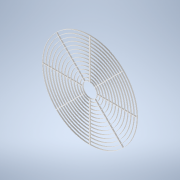
# Autodesk Inventor part: GitterUnten
Saved by Autodesk Inventor 2020.3 (Build 243373000, 373)
## iProperties
Created: 2020-08-06
Part Number: GitterUnten
Material: Generisch
Document SubType Name: Modeling
Designer: Stefan
Density: 1 g/cm^3
Appearance: Vorgabe
Author: Stefan
Autodesk Inventor part; units mm, degrees
ref_plane "YZ Plane" through (0, 0, 0) normal (1, 0, 0) x (0, 1, 0)
ref_plane "XZ Plane" through (0, 0, 0) normal (0, 1, 0) x (-1, 0, 0)
ref_plane "XY Plane" through (0, 0, 0) normal (0, 0, 1) x (1, 0, 0)
sketch "Skizze1" plane through (0, 0, 0) normal (0, 0, 1) x (1, 0, 0)
  line L0 (-278.3282, -259.073) -> (-259.0817, -278.3194) construction
  line L1 (-46.0536, -35.2636) -> (-10.8976, -70.4197) construction
  line L2 (-57.4999, 19.1327) -> (-57.4999, -6.5211) construction
  line L3 (-49.3128, 32.0045) -> (-8.1395, 73.1778) construction
  line L4 (-2, -377.9947) -> (-2, -354.9944)
  line L5 (-2, -352.9943) -> (-2, -329.9939)
  line L6 (-2, -327.9939) -> (-2, -304.9934)
  line L7 (-2, -302.9934) -> (-2, -279.9929)
  line L8 (-2, -277.9928) -> (-2, -254.9922)
  line L9 (-2, -252.9921) -> (-2, -229.9913)
  line L10 (-2, -227.9912) -> (-2, -204.9902)
  line L11 (-2, -202.9902) -> (-2, -179.9889)
  line L12 (-2, -177.9888) -> (-2, -154.9871)
  line L13 (-2, -152.9869) -> (-2, -129.9846)
  line L14 (-2, -127.9844) -> (-2, -104.981)
  line L15 (-2, -102.9806) -> (-2, -79.975)
  line L16 (-2, -77.9744) -> (-2, -59.4664)
  arc A0 (-265.8684, -268.6968) -> (-2, -377.9947) centre (0, 0) ccw
  arc A1 (-249.6047, -252.4331) -> (-2, -354.9944) centre (0, 0) ccw
  arc A2 (-248.1905, -251.0189) -> (-2, -352.9943) centre (0, 0) ccw
  line L17 (-252.4331, -249.6047) -> (-268.6968, -265.8684)
  line L18 (-265.8684, -268.6968) -> (-249.6047, -252.4331)
  arc A3 (-214.2487, -217.0771) -> (-2, -304.9934) centre (0, 0) ccw
  arc A4 (-212.8345, -215.6629) -> (-2, -302.9934) centre (0, 0) ccw
  arc A5 (-196.5706, -199.3991) -> (-2, -279.9929) centre (0, 0) ccw
  arc A6 (-178.8925, -181.7209) -> (-2, -254.9922) centre (0, 0) ccw
  arc A7 (-177.4782, -180.3066) -> (-2, -252.9921) centre (0, 0) ccw
  arc A8 (-161.2142, -164.0426) -> (-2, -229.9913) centre (0, 0) ccw
  arc A9 (-159.7999, -162.6284) -> (-2, -227.9912) centre (0, 0) ccw
  arc A10 (-143.5358, -146.3642) -> (-2, -204.9902) centre (0, 0) ccw
  arc A11 (-142.1215, -144.9499) -> (-2, -202.9902) centre (0, 0) ccw
  arc A12 (-231.9267, -234.7552) -> (-2, -329.9939) centre (0, 0) ccw
  arc A13 (-230.5125, -233.3409) -> (-2, -327.9939) centre (0, 0) ccw
  line L19 (-234.7552, -231.9267) -> (-251.0189, -248.1905)
  line L20 (-248.1905, -251.0189) -> (-231.9267, -234.7552)
  line L21 (-217.0771, -214.2487) -> (-233.3409, -230.5125)
  line L22 (-230.5125, -233.3409) -> (-214.2487, -217.0771)
  line L23 (-199.3991, -196.5706) -> (-215.6629, -212.8345)
  arc A14 (-195.1564, -197.9848) -> (-2, -277.9928) centre (0, 0) ccw
  line L24 (-212.8345, -215.6629) -> (-196.5706, -199.3991)
  line L25 (-181.7209, -178.8925) -> (-197.9848, -195.1564)
  line L26 (-195.1564, -197.9848) -> (-178.8925, -181.7209)
  line L27 (-164.0426, -161.2142) -> (-180.3066, -177.4782)
  line L28 (-177.4782, -180.3066) -> (-161.2142, -164.0426)
  line L29 (-146.3642, -143.5358) -> (-162.6284, -159.7999)
  line L30 (-159.7999, -162.6284) -> (-143.5358, -146.3642)
  arc A15 (-125.8572, -128.6856) -> (-2, -179.9889) centre (0, 0) ccw
  line L31 (-128.6856, -125.8572) -> (-144.9499, -142.1215)
  arc A16 (-124.4428, -127.2713) -> (-2, -177.9888) centre (0, 0) ccw
  line L32 (-142.1215, -144.9499) -> (-125.8572, -128.6856)
  arc A17 (-108.1782, -111.0066) -> (-2, -154.9871) centre (0, 0) ccw
  line L33 (-111.0066, -108.1782) -> (-127.2713, -124.4428)
  arc A18 (-106.7639, -109.5923) -> (-2, -152.9869) centre (0, 0) ccw
  line L34 (-124.4428, -127.2713) -> (-108.1782, -111.0066)
  arc A19 (-90.4988, -93.3272) -> (-2, -129.9846) centre (0, 0) ccw
  line L35 (-93.3272, -90.4988) -> (-109.5923, -106.7639)
  arc A20 (-89.0844, -91.9128) -> (-2, -127.9844) centre (0, 0) ccw
  line L36 (-106.7639, -109.5923) -> (-90.4988, -93.3272)
  arc A21 (-72.8185, -75.647) -> (-2, -104.981) centre (0, 0) ccw
  line L37 (-75.647, -72.8185) -> (-91.9128, -89.0844)
  line L38 (-89.0844, -91.9128) -> (-72.8185, -75.647)
  arc A22 (-71.4041, -74.2325) -> (-2, -102.9806) centre (0, 0) ccw
  arc A23 (-55.1366, -57.9651) -> (-2, -79.975) centre (0, 0) ccw
  line L39 (-43.4633, -40.6349) -> (-56.5504, -53.722)
  line L40 (-57.9651, -55.1366) -> (-74.2325, -71.4041)
  arc A24 (-53.722, -56.5504) -> (-2, -77.9744) centre (0, 0) ccw
  line L41 (-71.4041, -74.2325) -> (-55.1366, -57.9651)
  line L42 (-53.722, -56.5504) -> (-40.6349, -43.4633)
  arc A25 (-40.6349, -43.4633) -> (-2, -59.4664) centre (0, 0) ccw
  arc A26 (-377.9947, -2) -> (-268.6968, -265.8684) centre (0, 0) ccw
  arc A27 (-354.9944, -2) -> (-252.4331, -249.6047) centre (0, 0) ccw
  arc A28 (-352.9943, -2) -> (-251.0189, -248.1905) centre (0, 0) ccw
  arc A29 (-329.9939, -2) -> (-234.7552, -231.9267) centre (0, 0) ccw
  arc A30 (-327.9939, -2.0001) -> (-233.3409, -230.5125) centre (0, 0) ccw
  line L43 (-354.9944, -2) -> (-377.9947, -2)
  line L44 (-377.9947, 2) -> (-354.9944, 2)
  line L45 (-329.9939, -2) -> (-352.9943, -2)
  line L46 (-352.9943, 2) -> (-329.9939, 2)
  arc A31 (-304.9934, -2.0001) -> (-217.0771, -214.2487) centre (0, 0) ccw
  arc A32 (-302.9934, -2.0001) -> (-215.6629, -212.8345) centre (0, 0) ccw
  line L47 (-304.9934, -2.0001) -> (-327.9939, -2.0001)
  line L48 (-327.9939, 1.9999) -> (-304.9934, 1.9999)
  arc A33 (-279.9929, -2.0001) -> (-199.3991, -196.5706) centre (0, 0) ccw
  arc A34 (-277.9928, -2.0001) -> (-197.9848, -195.1564) centre (0, 0) ccw
  line L49 (-279.9929, -2.0001) -> (-302.9934, -2.0001)
  line L50 (-302.9934, 1.9999) -> (-279.9929, 1.9999)
  arc A35 (-254.9922, -2.0001) -> (-181.7209, -178.8925) centre (0, 0) ccw
  line L51 (-254.9922, -2.0001) -> (-277.9928, -2.0001)
  arc A36 (-252.9921, -2.0001) -> (-180.3066, -177.4782) centre (0, 0) ccw
  line L52 (-277.9928, 1.9999) -> (-254.9922, 1.9999)
  arc A37 (-229.9913, -2.0001) -> (-164.0426, -161.2142) centre (0, 0) ccw
  arc A38 (-227.9912, -2.0001) -> (-162.6284, -159.7999) centre (0, 0) ccw
  line L53 (-229.9913, -2.0001) -> (-252.9921, -2.0001)
  line L54 (-252.9921, 1.9999) -> (-229.9913, 1.9999)
  arc A39 (-204.9902, -2.0001) -> (-146.3642, -143.5358) centre (0, 0) ccw
  arc A40 (-202.9901, -2.0001) -> (-144.9499, -142.1215) centre (0, 0) ccw
  arc A41 (-179.9889, -2.0001) -> (-128.6856, -125.8572) centre (0, 0) ccw
  arc A42 (-177.9888, -2.0001) -> (-127.2713, -124.4428) centre (0, 0) ccw
  line L55 (-204.9902, -2.0001) -> (-227.9912, -2.0001)
  line L56 (-227.9912, 1.9999) -> (-204.9902, 1.9999)
  line L57 (-179.9889, -2.0001) -> (-202.9901, -2.0001)
  line L58 (-202.9901, 1.9999) -> (-179.9889, 1.9999)
  arc A43 (-154.9871, -2.0001) -> (-111.0066, -108.1782) centre (0, 0) ccw
  arc A44 (-152.9869, -2.0001) -> (-109.5923, -106.7639) centre (0, 0) ccw
  line L59 (-154.9871, -2.0001) -> (-177.9888, -2.0001)
  line L60 (-177.9888, 1.9999) -> (-154.9871, 1.9999)
  arc A45 (-129.9846, -2.0001) -> (-93.3272, -90.4988) centre (0, 0) ccw
  arc A46 (-127.9844, -2.0001) -> (-91.9128, -89.0844) centre (0, 0) ccw
  line L61 (-152.9869, 1.9999) -> (-129.9846, 1.9999)
  line L62 (-129.9846, -2.0001) -> (-152.9869, -2.0001)
  arc A47 (-104.9809, -2.0001) -> (-75.647, -72.8185) centre (0, 0) ccw
  arc A48 (-102.9806, -2.0001) -> (-74.2325, -71.4041) centre (0, 0) ccw
  arc A49 (-79.975, -2.0001) -> (-57.9651, -55.1366) centre (0, 0) ccw
  arc A50 (-77.9743, -2.0001) -> (-56.5504, -53.722) centre (0, 0) ccw
  line L63 (-104.9809, -2.0001) -> (-127.9844, -2.0001)
  line L64 (-127.9844, 1.9999) -> (-104.981, 1.9999)
  line L65 (-59.4664, -2.0001) -> (-77.9743, -2.0001)
  line L66 (-79.975, -2.0001) -> (-102.9806, -2.0001)
  line L67 (-102.9806, 1.9999) -> (-79.975, 1.9999)
  line L68 (-77.9743, 1.9999) -> (-59.4664, 1.9999)
  arc A51 (-59.4664, -2.0001) -> (-43.4633, -40.6349) centre (0, 0) ccw
  arc A52 (-43.4633, 40.6348) -> (-59.4664, 1.9999) centre (0, 0) ccw
  line L69 (-56.5504, 53.722) -> (-43.4633, 40.6348)
  arc A53 (-57.9651, 55.1366) -> (-79.975, 1.9999) centre (0, 0) ccw
  arc A54 (-56.5504, 53.722) -> (-77.9743, 1.9999) centre (0, 0) ccw
  line L70 (-40.6349, 43.4633) -> (-53.722, 56.5504)
  line L71 (-74.2325, 71.404) -> (-57.9651, 55.1366)
  line L72 (-55.1367, 57.9651) -> (-71.4041, 74.2325)
  arc A55 (-75.647, 72.8185) -> (-104.981, 1.9999) centre (0, 0) ccw
  arc A56 (-74.2325, 71.404) -> (-102.9806, 1.9999) centre (0, 0) ccw
  line L73 (-91.9128, 89.0844) -> (-75.647, 72.8185)
  line L74 (-72.8185, 75.6469) -> (-89.0844, 91.9128)
  arc A57 (-91.9128, 89.0844) -> (-127.9844, 1.9999) centre (0, 0) ccw
  arc A58 (-93.3272, 90.4988) -> (-129.9846, 1.9999) centre (0, 0) ccw
  line L75 (-109.5923, 106.7639) -> (-93.3272, 90.4988)
  arc A59 (-111.0067, 108.1782) -> (-154.9871, 1.9999) centre (0, 0) ccw
  line L76 (-90.4988, 93.3272) -> (-106.7639, 109.5923)
  arc A60 (-109.5923, 106.7639) -> (-152.9869, 1.9999) centre (0, 0) ccw
  line L77 (-127.2713, 124.4428) -> (-111.0067, 108.1782)
  line L78 (-108.1782, 111.0066) -> (-124.4429, 127.2712)
  arc A61 (-127.2713, 124.4428) -> (-177.9888, 1.9999) centre (0, 0) ccw
  arc A62 (-128.6856, 125.8571) -> (-179.9889, 1.9999) centre (0, 0) ccw
  arc A63 (-162.6284, 159.7999) -> (-227.9912, 1.9999) centre (0, 0) ccw
  arc A64 (-164.0427, 161.2142) -> (-229.9913, 1.9999) centre (0, 0) ccw
  arc A65 (-146.3642, 143.5357) -> (-204.9902, 1.9999) centre (0, 0) ccw
  arc A66 (-144.9499, 142.1215) -> (-202.9901, 1.9999) centre (0, 0) ccw
  line L79 (-162.6284, 159.7999) -> (-146.3642, 143.5357)
  line L80 (-144.9499, 142.1215) -> (-128.6856, 125.8571)
  line L81 (-125.8572, 128.6856) -> (-142.1215, 144.9499)
  line L82 (-143.5358, 146.3642) -> (-159.7999, 162.6283)
  arc A67 (-180.3067, 177.4782) -> (-252.9921, 1.9999) centre (0, 0) ccw
  arc A68 (-181.7209, 178.8924) -> (-254.9922, 1.9999) centre (0, 0) ccw
  arc A69 (-197.9848, 195.1563) -> (-277.9928, 1.9999) centre (0, 0) ccw
  arc A70 (-199.3991, 196.5706) -> (-279.9929, 1.9999) centre (0, 0) ccw
  arc A71 (-215.6629, 212.8344) -> (-302.9934, 1.9999) centre (0, 0) ccw
  arc A72 (-217.0772, 214.2487) -> (-304.9934, 1.9999) centre (0, 0) ccw
  arc A73 (-251.0189, 248.1904) -> (-352.9943, 2) centre (0, 0) ccw
  arc A74 (-252.4332, 249.6047) -> (-354.9944, 2) centre (0, 0) ccw
  arc A75 (-234.7552, 231.9267) -> (-329.9939, 2) centre (0, 0) ccw
  arc A76 (-233.3409, 230.5124) -> (-327.9939, 1.9999) centre (0, 0) ccw
  line L83 (-251.0189, 248.1904) -> (-234.7552, 231.9267)
  line L84 (-231.9268, 234.7551) -> (-248.1905, 251.0188)
  line L85 (-233.3409, 230.5124) -> (-217.0772, 214.2487)
  line L86 (-214.2488, 217.0771) -> (-230.5125, 233.3409)
  line L87 (-215.6629, 212.8344) -> (-199.3991, 196.5706)
  line L88 (-196.5707, 199.399) -> (-212.8345, 215.6629)
  line L89 (-197.9848, 195.1563) -> (-181.7209, 178.8924)
  line L90 (-180.3067, 177.4782) -> (-164.0427, 161.2142)
  line L91 (-161.2142, 164.0426) -> (-177.4782, 180.3066)
  line L92 (-178.8925, 181.7209) -> (-195.1564, 197.9848)
  line L93 (-268.6969, 265.8684) -> (-252.4332, 249.6047)
  arc A77 (-268.6969, 265.8684) -> (-377.9947, 2) centre (0, 0) ccw
  line L94 (-249.6047, 252.4331) -> (-265.8684, 268.6968)
  arc A78 (-2, 377.9947) -> (-265.8684, 268.6968) centre (0, 0) ccw
  line L95 (-2, 377.9947) -> (-2, 354.9944)
  line L96 (-2, 377.9947) -> (-2, 354.9944)
  arc A79 (-2, 352.9943) -> (-248.1905, 251.0188) centre (0, 0) ccw
  arc A80 (-2, 354.9944) -> (-249.6047, 252.4331) centre (0, 0) ccw
  line L97 (-2, 352.9943) -> (-2, 329.9939)
  line L98 (-2, 352.9943) -> (-2, 329.9939)
  arc A81 (-2, 327.9939) -> (-230.5125, 233.3409) centre (0, 0) ccw
  arc A82 (-2, 329.9939) -> (-231.9268, 234.7551) centre (0, 0) ccw
  arc A83 (-2, 304.9934) -> (-214.2488, 217.0771) centre (0, 0) ccw
  arc A84 (-2, 302.9934) -> (-212.8345, 215.6629) centre (0, 0) ccw
  line L99 (-2, 327.9939) -> (-2, 304.9934)
  line L100 (-2, 327.9939) -> (-2, 304.9934)
  arc A85 (-2, 279.9929) -> (-196.5707, 199.399) centre (0, 0) ccw
  arc A86 (-2, 277.9928) -> (-195.1564, 197.9848) centre (0, 0) ccw
  line L101 (-2, 302.9934) -> (-2, 279.9929)
  line L102 (-2, 302.9934) -> (-2, 279.9929)
  arc A87 (-2, 254.9922) -> (-178.8925, 181.7209) centre (0, 0) ccw
  arc A88 (-2, 252.9921) -> (-177.4782, 180.3066) centre (0, 0) ccw
  line L103 (-2, 277.9928) -> (-2, 254.9922)
  line L104 (-2, 277.9928) -> (-2, 254.9922)
  line L105 (-2, 252.9921) -> (-2, 229.9913)
  line L106 (-2, 252.9921) -> (-2, 229.9913)
  arc A89 (-2, 227.9912) -> (-159.7999, 162.6283) centre (0, 0) ccw
  arc A90 (-2, 229.9913) -> (-161.2142, 164.0426) centre (0, 0) ccw
  arc A91 (-2, 202.9901) -> (-142.1215, 144.9499) centre (0, 0) ccw
  arc A92 (-2, 204.9902) -> (-143.5358, 146.3642) centre (0, 0) ccw
  line L107 (-2, 227.9912) -> (-2, 204.9902)
  line L108 (-2, 227.9912) -> (-2, 204.9902)
  arc A93 (-2, 179.9889) -> (-125.8572, 128.6856) centre (0, 0) ccw
  arc A94 (-2, 177.9888) -> (-124.4429, 127.2712) centre (0, 0) ccw
  line L109 (-2, 202.9901) -> (-2, 179.9889)
  line L110 (-2, 202.9901) -> (-2, 179.9889)
  arc A95 (-2, 154.9871) -> (-108.1782, 111.0066) centre (0, 0) ccw
  arc A96 (-2, 152.9869) -> (-106.7639, 109.5923) centre (0, 0) ccw
  line L111 (-2, 177.9888) -> (-2, 154.9871)
  line L112 (-2, 177.9888) -> (-2, 154.9871)
  arc A97 (-2, 129.9846) -> (-90.4988, 93.3272) centre (0, 0) ccw
  arc A98 (-2, 127.9844) -> (-89.0844, 91.9128) centre (0, 0) ccw
  arc A99 (-2, 104.981) -> (-72.8185, 75.6469) centre (0, 0) ccw
  arc A100 (-2, 102.9806) -> (-71.4041, 74.2325) centre (0, 0) ccw
  arc A101 (-2, 79.975) -> (-55.1367, 57.9651) centre (0, 0) ccw
  line L113 (-2, 152.9869) -> (-2, 129.9846)
  line L114 (-2, 152.9869) -> (-2, 129.9846)
  line L115 (-2, 127.9844) -> (-2, 104.981)
  line L116 (-2, 127.9844) -> (-2, 104.981)
  arc A102 (-2, 77.9743) -> (-53.722, 56.5504) centre (0, 0) ccw
  line L117 (-2, 102.9806) -> (-2, 79.975)
  line L118 (-2, 77.9743) -> (-2, 59.4664)
  line L119 (-2, 102.9806) -> (-2, 79.975)
  line L120 (-2, 77.9743) -> (-2, 59.4664)
  arc A103 (-2, 59.4664) -> (-40.6349, 43.4633) centre (0, 0) ccw
  line L121 (0, -447.5896) -> (0, 831.5274) construction
  arc A104 (0, 57.5) -> (0, -57.5) centre (0, 0) ccw
  arc A105 (0, 380) -> (0, -380) centre (0, 0) ccw
  line L122 (278.3282, -259.073) -> (259.0817, -278.3194) construction
  line L123 (46.0536, -35.2636) -> (10.8976, -70.4197) construction
  line L124 (57.4999, 19.1327) -> (57.4999, -6.5211) construction
  line L125 (49.3128, 32.0045) -> (8.1395, 73.1778) construction
  line L126 (2, -377.9947) -> (2, -354.9944)
  line L127 (2, -352.9943) -> (2, -329.9939)
  line L128 (2, -327.9939) -> (2, -304.9934)
  line L129 (2, -302.9934) -> (2, -279.9929)
  line L130 (2, -277.9928) -> (2, -254.9922)
  line L131 (2, -252.9921) -> (2, -229.9913)
  line L132 (2, -227.9912) -> (2, -204.9902)
  line L133 (2, -202.9902) -> (2, -179.9889)
  line L134 (2, -177.9888) -> (2, -154.9871)
  line L135 (2, -152.9869) -> (2, -129.9846)
  line L136 (2, -127.9844) -> (2, -104.981)
  line L137 (2, -102.9806) -> (2, -79.975)
  line L138 (2, -77.9744) -> (2, -59.4664)
  arc A106 (2, -377.9947) -> (265.8684, -268.6968) centre (0, 0) ccw
  arc A107 (2, -354.9944) -> (249.6047, -252.4331) centre (0, 0) ccw
  arc A108 (2, -352.9943) -> (248.1905, -251.0189) centre (0, 0) ccw
  line L139 (252.4331, -249.6047) -> (268.6968, -265.8684)
  line L140 (265.8684, -268.6968) -> (249.6047, -252.4331)
  arc A109 (2, -304.9934) -> (214.2487, -217.0771) centre (0, 0) ccw
  arc A110 (2, -302.9934) -> (212.8345, -215.6629) centre (0, 0) ccw
  arc A111 (2, -279.9929) -> (196.5706, -199.3991) centre (0, 0) ccw
  arc A112 (2, -254.9922) -> (178.8925, -181.7209) centre (0, 0) ccw
  arc A113 (2, -252.9921) -> (177.4782, -180.3066) centre (0, 0) ccw
  arc A114 (2, -229.9913) -> (161.2142, -164.0426) centre (0, 0) ccw
  arc A115 (2, -227.9912) -> (159.7999, -162.6284) centre (0, 0) ccw
  arc A116 (2, -204.9902) -> (143.5358, -146.3642) centre (0, 0) ccw
  arc A117 (2, -202.9902) -> (142.1215, -144.9499) centre (0, 0) ccw
  arc A118 (2, -329.9939) -> (231.9267, -234.7552) centre (0, 0) ccw
  arc A119 (2, -327.9939) -> (230.5125, -233.3409) centre (0, 0) ccw
  line L141 (234.7552, -231.9267) -> (251.0189, -248.1905)
  line L142 (248.1905, -251.0189) -> (231.9267, -234.7552)
  line L143 (217.0771, -214.2487) -> (233.3409, -230.5125)
  line L144 (230.5125, -233.3409) -> (214.2487, -217.0771)
  line L145 (199.3991, -196.5706) -> (215.6629, -212.8345)
  arc A120 (2, -277.9928) -> (195.1564, -197.9848) centre (0, 0) ccw
  line L146 (212.8345, -215.6629) -> (196.5706, -199.3991)
  line L147 (181.7209, -178.8925) -> (197.9848, -195.1564)
  line L148 (195.1564, -197.9848) -> (178.8925, -181.7209)
  line L149 (164.0426, -161.2142) -> (180.3066, -177.4782)
  line L150 (177.4782, -180.3066) -> (161.2142, -164.0426)
  line L151 (146.3642, -143.5358) -> (162.6284, -159.7999)
  line L152 (159.7999, -162.6284) -> (143.5358, -146.3642)
  arc A121 (2, -179.9889) -> (125.8572, -128.6856) centre (0, 0) ccw
  line L153 (128.6856, -125.8572) -> (144.9499, -142.1215)
  arc A122 (2, -177.9888) -> (124.4428, -127.2713) centre (0, 0) ccw
  line L154 (142.1215, -144.9499) -> (125.8572, -128.6856)
  arc A123 (2, -154.9871) -> (108.1782, -111.0066) centre (0, 0) ccw
  line L155 (111.0066, -108.1782) -> (127.2713, -124.4428)
  arc A124 (2, -152.9869) -> (106.7639, -109.5923) centre (0, 0) ccw
  line L156 (124.4428, -127.2713) -> (108.1782, -111.0066)
  arc A125 (2, -129.9846) -> (90.4988, -93.3272) centre (0, 0) ccw
  line L157 (93.3272, -90.4988) -> (109.5923, -106.7639)
  arc A126 (2, -127.9844) -> (89.0844, -91.9128) centre (0, 0) ccw
  line L158 (106.7639, -109.5923) -> (90.4988, -93.3272)
  arc A127 (2, -104.981) -> (72.8185, -75.647) centre (0, 0) ccw
  line L159 (75.647, -72.8185) -> (91.9128, -89.0844)
  line L160 (89.0844, -91.9128) -> (72.8185, -75.647)
  arc A128 (2, -102.9806) -> (71.4041, -74.2325) centre (0, 0) ccw
  arc A129 (2, -79.975) -> (55.1366, -57.9651) centre (0, 0) ccw
  line L161 (43.4633, -40.6349) -> (56.5504, -53.722)
  line L162 (57.9651, -55.1366) -> (74.2325, -71.4041)
  arc A130 (2, -77.9744) -> (53.722, -56.5504) centre (0, 0) ccw
  line L163 (71.4041, -74.2325) -> (55.1366, -57.9651)
  line L164 (53.722, -56.5504) -> (40.6349, -43.4633)
  arc A131 (2, -59.4664) -> (40.6349, -43.4633) centre (0, 0) ccw
  arc A132 (268.6968, -265.8684) -> (377.9947, -2) centre (0, 0) ccw
  arc A133 (252.4331, -249.6047) -> (354.9944, -2) centre (0, 0) ccw
  arc A134 (251.0189, -248.1905) -> (352.9943, -2) centre (0, 0) ccw
  arc A135 (234.7552, -231.9267) -> (329.9939, -2) centre (0, 0) ccw
  arc A136 (233.3409, -230.5125) -> (327.9939, -2.0001) centre (0, 0) ccw
  line L165 (354.9944, -2) -> (377.9947, -2)
  line L166 (377.9947, 2) -> (354.9944, 2)
  line L167 (329.9939, -2) -> (352.9943, -2)
  line L168 (352.9943, 2) -> (329.9939, 2)
  arc A137 (217.0771, -214.2487) -> (304.9934, -2.0001) centre (0, 0) ccw
  arc A138 (215.6629, -212.8345) -> (302.9934, -2.0001) centre (0, 0) ccw
  line L169 (304.9934, -2.0001) -> (327.9939, -2.0001)
  line L170 (327.9939, 1.9999) -> (304.9934, 1.9999)
  arc A139 (199.3991, -196.5706) -> (279.9929, -2.0001) centre (0, 0) ccw
  arc A140 (197.9848, -195.1564) -> (277.9928, -2.0001) centre (0, 0) ccw
  line L171 (279.9929, -2.0001) -> (302.9934, -2.0001)
  line L172 (302.9934, 1.9999) -> (279.9929, 1.9999)
  arc A141 (181.7209, -178.8925) -> (254.9922, -2.0001) centre (0, 0) ccw
  line L173 (254.9922, -2.0001) -> (277.9928, -2.0001)
  arc A142 (180.3066, -177.4782) -> (252.9921, -2.0001) centre (0, 0) ccw
  line L174 (277.9928, 1.9999) -> (254.9922, 1.9999)
  arc A143 (164.0426, -161.2142) -> (229.9913, -2.0001) centre (0, 0) ccw
  arc A144 (162.6284, -159.7999) -> (227.9912, -2.0001) centre (0, 0) ccw
  line L175 (229.9913, -2.0001) -> (252.9921, -2.0001)
  line L176 (252.9921, 1.9999) -> (229.9913, 1.9999)
  arc A145 (146.3642, -143.5358) -> (204.9902, -2.0001) centre (0, 0) ccw
  arc A146 (144.9499, -142.1215) -> (202.9901, -2.0001) centre (0, 0) ccw
  arc A147 (128.6856, -125.8572) -> (179.9889, -2.0001) centre (0, 0) ccw
  arc A148 (127.2713, -124.4428) -> (177.9888, -2.0001) centre (0, 0) ccw
  line L177 (204.9902, -2.0001) -> (227.9912, -2.0001)
  line L178 (227.9912, 1.9999) -> (204.9902, 1.9999)
  line L179 (179.9889, -2.0001) -> (202.9901, -2.0001)
  line L180 (202.9901, 1.9999) -> (179.9889, 1.9999)
  arc A149 (111.0066, -108.1782) -> (154.9871, -2.0001) centre (0, 0) ccw
  arc A150 (109.5923, -106.7639) -> (152.9869, -2.0001) centre (0, 0) ccw
  line L181 (154.9871, -2.0001) -> (177.9888, -2.0001)
  line L182 (177.9888, 1.9999) -> (154.9871, 1.9999)
  arc A151 (93.3272, -90.4988) -> (129.9846, -2.0001) centre (0, 0) ccw
  arc A152 (91.9128, -89.0844) -> (127.9844, -2.0001) centre (0, 0) ccw
  line L183 (152.9869, 1.9999) -> (129.9846, 1.9999)
  line L184 (129.9846, -2.0001) -> (152.9869, -2.0001)
  arc A153 (75.647, -72.8185) -> (104.9809, -2.0001) centre (0, 0) ccw
  arc A154 (74.2325, -71.4041) -> (102.9806, -2.0001) centre (0, 0) ccw
  arc A155 (57.9651, -55.1366) -> (79.975, -2.0001) centre (0, 0) ccw
  arc A156 (56.5504, -53.722) -> (77.9743, -2.0001) centre (0, 0) ccw
  line L185 (104.9809, -2.0001) -> (127.9844, -2.0001)
  line L186 (127.9844, 1.9999) -> (104.981, 1.9999)
  line L187 (59.4664, -2.0001) -> (77.9743, -2.0001)
  line L188 (79.975, -2.0001) -> (102.9806, -2.0001)
  line L189 (102.9806, 1.9999) -> (79.975, 1.9999)
  line L190 (77.9743, 1.9999) -> (59.4664, 1.9999)
  arc A157 (43.4633, -40.6349) -> (59.4664, -2.0001) centre (0, 0) ccw
  arc A158 (59.4664, 1.9999) -> (43.4633, 40.6348) centre (0, 0) ccw
  line L191 (56.5504, 53.722) -> (43.4633, 40.6348)
  arc A159 (79.975, 1.9999) -> (57.9651, 55.1366) centre (0, 0) ccw
  arc A160 (77.9743, 1.9999) -> (56.5504, 53.722) centre (0, 0) ccw
  line L192 (40.6349, 43.4633) -> (53.722, 56.5504)
  line L193 (74.2325, 71.404) -> (57.9651, 55.1366)
  line L194 (55.1367, 57.9651) -> (71.4041, 74.2325)
  arc A161 (104.981, 1.9999) -> (75.647, 72.8185) centre (0, 0) ccw
  arc A162 (102.9806, 1.9999) -> (74.2325, 71.404) centre (0, 0) ccw
  line L195 (91.9128, 89.0844) -> (75.647, 72.8185)
  line L196 (72.8185, 75.6469) -> (89.0844, 91.9128)
  arc A163 (127.9844, 1.9999) -> (91.9128, 89.0844) centre (0, 0) ccw
  arc A164 (129.9846, 1.9999) -> (93.3272, 90.4988) centre (0, 0) ccw
  line L197 (109.5923, 106.7639) -> (93.3272, 90.4988)
  arc A165 (154.9871, 1.9999) -> (111.0067, 108.1782) centre (0, 0) ccw
  line L198 (90.4988, 93.3272) -> (106.7639, 109.5923)
  arc A166 (152.9869, 1.9999) -> (109.5923, 106.7639) centre (0, 0) ccw
  line L199 (127.2713, 124.4428) -> (111.0067, 108.1782)
  line L200 (108.1782, 111.0066) -> (124.4429, 127.2712)
  arc A167 (177.9888, 1.9999) -> (127.2713, 124.4428) centre (0, 0) ccw
  arc A168 (179.9889, 1.9999) -> (128.6856, 125.8571) centre (0, 0) ccw
  arc A169 (227.9912, 1.9999) -> (162.6284, 159.7999) centre (0, 0) ccw
  arc A170 (229.9913, 1.9999) -> (164.0427, 161.2142) centre (0, 0) ccw
  arc A171 (204.9902, 1.9999) -> (146.3642, 143.5357) centre (0, 0) ccw
  arc A172 (202.9901, 1.9999) -> (144.9499, 142.1215) centre (0, 0) ccw
  line L201 (162.6284, 159.7999) -> (146.3642, 143.5357)
  line L202 (144.9499, 142.1215) -> (128.6856, 125.8571)
  line L203 (125.8572, 128.6856) -> (142.1215, 144.9499)
  line L204 (143.5358, 146.3642) -> (159.7999, 162.6283)
  arc A173 (252.9921, 1.9999) -> (180.3067, 177.4782) centre (0, 0) ccw
  arc A174 (254.9922, 1.9999) -> (181.7209, 178.8924) centre (0, 0) ccw
  arc A175 (277.9928, 1.9999) -> (197.9848, 195.1563) centre (0, 0) ccw
  arc A176 (279.9929, 1.9999) -> (199.3991, 196.5706) centre (0, 0) ccw
  arc A177 (302.9934, 1.9999) -> (215.6629, 212.8344) centre (0, 0) ccw
  arc A178 (304.9934, 1.9999) -> (217.0772, 214.2487) centre (0, 0) ccw
  arc A179 (352.9943, 2) -> (251.0189, 248.1904) centre (0, 0) ccw
  arc A180 (354.9944, 2) -> (252.4332, 249.6047) centre (0, 0) ccw
  arc A181 (329.9939, 2) -> (234.7552, 231.9267) centre (0, 0) ccw
  arc A182 (327.9939, 1.9999) -> (233.3409, 230.5124) centre (0, 0) ccw
  line L205 (251.0189, 248.1904) -> (234.7552, 231.9267)
  line L206 (231.9268, 234.7551) -> (248.1905, 251.0188)
  line L207 (233.3409, 230.5124) -> (217.0772, 214.2487)
  line L208 (214.2488, 217.0771) -> (230.5125, 233.3409)
  line L209 (215.6629, 212.8344) -> (199.3991, 196.5706)
  line L210 (196.5707, 199.399) -> (212.8345, 215.6629)
  line L211 (197.9848, 195.1563) -> (181.7209, 178.8924)
  line L212 (180.3067, 177.4782) -> (164.0427, 161.2142)
  line L213 (161.2142, 164.0426) -> (177.4782, 180.3066)
  line L214 (178.8925, 181.7209) -> (195.1564, 197.9848)
  line L215 (268.6969, 265.8684) -> (252.4332, 249.6047)
  arc A183 (377.9947, 2) -> (268.6969, 265.8684) centre (0, 0) ccw
  line L216 (249.6047, 252.4331) -> (265.8684, 268.6968)
  arc A184 (265.8684, 268.6968) -> (2, 377.9947) centre (0, 0) ccw
  line L217 (2, 377.9947) -> (2, 354.9944)
  line L218 (2, 377.9947) -> (2, 354.9944)
  arc A185 (248.1905, 251.0188) -> (2, 352.9943) centre (0, 0) ccw
  arc A186 (249.6047, 252.4331) -> (2, 354.9944) centre (0, 0) ccw
  line L219 (2, 352.9943) -> (2, 329.9939)
  line L220 (2, 352.9943) -> (2, 329.9939)
  arc A187 (230.5125, 233.3409) -> (2, 327.9939) centre (0, 0) ccw
  arc A188 (231.9268, 234.7551) -> (2, 329.9939) centre (0, 0) ccw
  arc A189 (214.2488, 217.0771) -> (2, 304.9934) centre (0, 0) ccw
  arc A190 (212.8345, 215.6629) -> (2, 302.9934) centre (0, 0) ccw
  line L221 (2, 327.9939) -> (2, 304.9934)
  line L222 (2, 327.9939) -> (2, 304.9934)
  arc A191 (196.5707, 199.399) -> (2, 279.9929) centre (0, 0) ccw
  arc A192 (195.1564, 197.9848) -> (2, 277.9928) centre (0, 0) ccw
  line L223 (2, 302.9934) -> (2, 279.9929)
  line L224 (2, 302.9934) -> (2, 279.9929)
  arc A193 (178.8925, 181.7209) -> (2, 254.9922) centre (0, 0) ccw
  arc A194 (177.4782, 180.3066) -> (2, 252.9921) centre (0, 0) ccw
  line L225 (2, 277.9928) -> (2, 254.9922)
  line L226 (2, 277.9928) -> (2, 254.9922)
  line L227 (2, 252.9921) -> (2, 229.9913)
  line L228 (2, 252.9921) -> (2, 229.9913)
  arc A195 (159.7999, 162.6283) -> (2, 227.9912) centre (0, 0) ccw
  arc A196 (161.2142, 164.0426) -> (2, 229.9913) centre (0, 0) ccw
  arc A197 (142.1215, 144.9499) -> (2, 202.9901) centre (0, 0) ccw
  arc A198 (143.5358, 146.3642) -> (2, 204.9902) centre (0, 0) ccw
  line L229 (2, 227.9912) -> (2, 204.9902)
  line L230 (2, 227.9912) -> (2, 204.9902)
  arc A199 (125.8572, 128.6856) -> (2, 179.9889) centre (0, 0) ccw
  arc A200 (124.4429, 127.2712) -> (2, 177.9888) centre (0, 0) ccw
  line L231 (2, 202.9901) -> (2, 179.9889)
  line L232 (2, 202.9901) -> (2, 179.9889)
  arc A201 (108.1782, 111.0066) -> (2, 154.9871) centre (0, 0) ccw
  arc A202 (106.7639, 109.5923) -> (2, 152.9869) centre (0, 0) ccw
  line L233 (2, 177.9888) -> (2, 154.9871)
  line L234 (2, 177.9888) -> (2, 154.9871)
  arc A203 (90.4988, 93.3272) -> (2, 129.9846) centre (0, 0) ccw
  arc A204 (89.0844, 91.9128) -> (2, 127.9844) centre (0, 0) ccw
  arc A205 (72.8185, 75.6469) -> (2, 104.981) centre (0, 0) ccw
  arc A206 (71.4041, 74.2325) -> (2, 102.9806) centre (0, 0) ccw
  arc A207 (55.1367, 57.9651) -> (2, 79.975) centre (0, 0) ccw
  line L235 (2, 152.9869) -> (2, 129.9846)
  line L236 (2, 152.9869) -> (2, 129.9846)
  line L237 (2, 127.9844) -> (2, 104.981)
  line L238 (2, 127.9844) -> (2, 104.981)
  arc A208 (53.722, 56.5504) -> (2, 77.9743) centre (0, 0) ccw
  line L239 (2, 102.9806) -> (2, 79.975)
  line L240 (2, 77.9743) -> (2, 59.4664)
  line L241 (2, 102.9806) -> (2, 79.975)
  line L242 (2, 77.9743) -> (2, 59.4664)
  arc A209 (40.6349, 43.4633) -> (2, 59.4664) centre (0, 0) ccw
  arc A210 (0, -57.5) -> (0, 57.5) centre (0, 0) ccw
  arc A211 (0, -380) -> (0, 380) centre (0, 0) ccw
  point P0 (0, 0)
  point P1 (0, 57.5)
  constraints: 507 parallel, 486 end point, 424 point on circle, 239 symmetric about line, 212 centre point, 42 coincident, 3 point on line, 106 other
extrude "Extrusion1" add sketch "Skizze1" along normal blind 10
equation "\"dicke\" = 4"
equation "\"d30\" = dicke"
equation "\"d32\" = 0.5 * dicke"
equation "\"d33\" = 0.5 * dicke"
equation "\"d34\" = dicke"
equation "\"d36\" = dicke"
equation "\"d37\" = 0.5 * dicke"
equation "\"d39\" = 0.5 * dicke"
equation "\"d40\" = dicke"
equation "\"d41\" = 0.5 * dicke"
equation "\"d45\" = 0.5 * dicke"
equation "\"d49\" = dicke"
equation "\"d50\" = 0.5 * dicke"
